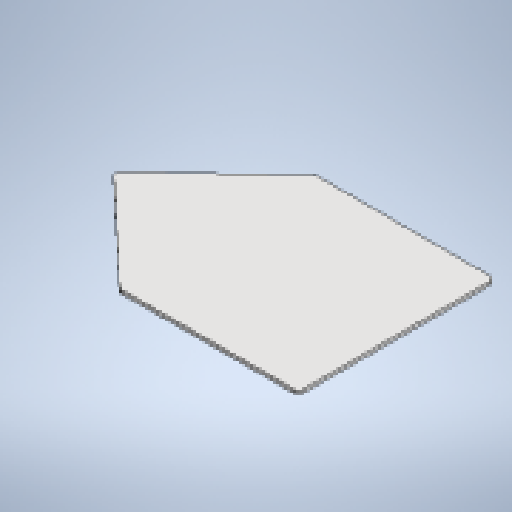
# Autodesk Inventor part: DS-B-502 CAPhouse
Saved by Autodesk Inventor 2025.1 (Build 291241020, 241B)
## iProperties
Created: 2025-01-16
Part Number: DS-B-502 CAPhouse
Material: Stainless Steel
Document SubType Name: Sheet Metal
Designer: pokla
Density: 8 g/cm^3
Sheet Metal Rule: AISI304 2mm Die16
Appearance: Default
Flat Pattern Width: 4.5 cm
Flat Pattern Length: 6.45379 cm
Flat Pattern Area: 29.042 cm^2
Sheet Metal Width: 45.000 mm
Sheet Metal Length: 64.538 mm
Sheet Metal Area: 2904.205 mm^2
Author: pokla
Autodesk Inventor part; units mm, degrees
ref_plane "YZ Plane" through (0, 0, 0) normal (1, 0, 0) x (0, 1, 0)
ref_plane "XZ Plane" through (0, 0, 0) normal (0, 1, 0) x (-1, 0, 0)
ref_plane "XY Plane" through (0, 0, 0) normal (0, 0, 1) x (1, 0, 0)
sketch "Sketch1" plane through (0, 0, 0) normal (0, 0, 1) x (1, 0, 0)
  line L0 (-20.5, 22.5) -> (20.5, 22.5)
  line L1 (20.5, 22.5) -> (20.5, -22.5)
  line L2 (20.5, -22.5) -> (-20.5, -22.5)
  line L3 (-20.5, -22.5) -> (-20.5, 22.5) construction
  line L4 (-20.5, 22.5) -> (20.5, -22.5) construction
  line L5 (-20.5, -22.5) -> (-44.5, 0)
  line L6 (-44.5, 0) -> (-20.5, 22.5)
  point P0 (0, 0)
  point P1 (0, 0)
  point P2 (20.5, 0)
  dimension "d0" = 41
  dimension "d1" = 45
  dimension "d4" = 65
  measures "d0" distance of L0.start L0.end
  measures "d1" distance of L2.end L0.start
  measures "d4" distance of point (20.5, 0) L5.end
extrude "Plate1" add sketch "Sketch1" along normal blind 0.8
fillet "Corner Round2" radius 1 5 edges at (-20.5, -22.5, 0.4) (-44.5, 0, 0.4) (-20.5, 22.5, 0.4) (20.5, -22.5, 0.4) (20.5, 22.5, 0.4)
equation "\"d2\" = Thickness"
equation "\"BendReliefWidth\" = Thickness"
equation "\"BendReliefDepth\" = 0.5 * Thickness"
equation "\"CornerReliefSize\" = 4 * Thickness"
equation "\"MinimumRemnant\" = 2 * Thickness"
equation "\"TransitionRadius\" = BendRadius"
equation "\"JacobiRadiusSize\" = BendRadius"
equation "\"GapSize\" = Thickness"
equation "\"Thickness\" = 0.8"
equation "\"BendRadius\" = 2.75"
body "Solid1"
